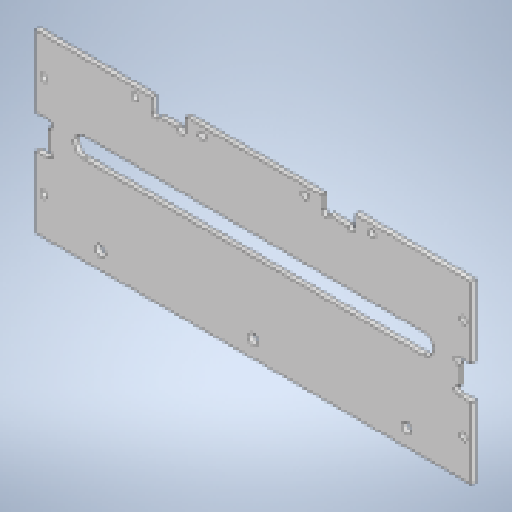
# Autodesk Inventor part: side_ita
Saved by Autodesk Inventor 2024 (Build 280153000, 153)
## iProperties
Created: 2024-06-05
Part Number: side_ita
Material: アルミニウム 2014-T4
Document SubType Name: Modeling
Designer: right
Density: 2.8 g/cm^3
Appearance: サテン
Author: right
Autodesk Inventor part; units mm, degrees
ref_plane "YZ Plane" through (0, 0, 0) normal (1, 0, 0) x (0, 1, 0)
ref_plane "XZ Plane" through (0, 0, 0) normal (0, 1, 0) x (-1, 0, 0)
ref_plane "XY Plane" through (0, 0, 0) normal (0, 0, 1) x (1, 0, 0)
sketch "スケッチ1" plane through (0, 0, 0) normal (0, 0, 1) x (1, 0, 0)
  line L0 (-50.5, 0.75) -> (50.5, 0.75) projected
  line L1 (50.5, 0.75) -> (50.5, 15.0295) projected
  line L2 (50.5, 15.0295) -> (49.637, 17.5) projected
  line L3 (49.637, 17.5) -> (47.2832, 17.5) projected
  line L4 (47.2832, 17.5) -> (44.9252, 10.75) projected
  line L5 (44.9252, 10.75) -> (42.5702, 10.75) projected
  line L6 (42.5702, 10.75) -> (40.2122, 17.5) projected
  line L7 (40.2122, 17.5) -> (37.8584, 17.5) projected
  line L8 (37.8584, 17.5) -> (35.5004, 10.75) projected
  line L9 (35.5004, 10.75) -> (33.1454, 10.75) projected
  line L10 (33.1454, 10.75) -> (30.7874, 17.5) projected
  line L11 (30.7874, 17.5) -> (28.4337, 17.5) projected
  line L12 (28.4337, 17.5) -> (26.0757, 10.75) projected
  line L13 (26.0757, 10.75) -> (23.7207, 10.75) projected
  line L14 (23.7207, 10.75) -> (21.3627, 17.5) projected
  line L15 (21.3627, 17.5) -> (19.0089, 17.5) projected
  line L16 (19.0089, 17.5) -> (16.6509, 10.75) projected
  line L17 (16.6509, 10.75) -> (14.2959, 10.75) projected
  line L18 (14.2959, 10.75) -> (11.9379, 17.5) projected
  line L19 (11.9379, 17.5) -> (9.5841, 17.5) projected
  line L20 (9.5841, 17.5) -> (7.2261, 10.75) projected
  line L21 (7.2261, 10.75) -> (4.8711, 10.75) projected
  line L22 (4.8711, 10.75) -> (2.5131, 17.5) projected
  line L23 (2.5131, 17.5) -> (0.1594, 17.5) projected
  line L24 (0.1594, 17.5) -> (-2.1986, 10.75) projected
  line L25 (-2.1986, 10.75) -> (-4.5536, 10.75) projected
  line L26 (-4.5536, 10.75) -> (-6.9116, 17.5) projected
  line L27 (-6.9116, 17.5) -> (-9.2654, 17.5) projected
  line L28 (-9.2654, 17.5) -> (-11.6234, 10.75) projected
  line L29 (-11.6234, 10.75) -> (-13.9784, 10.75) projected
  line L30 (-13.9784, 10.75) -> (-16.3364, 17.5) projected
  line L31 (-16.3364, 17.5) -> (-18.6902, 17.5) projected
  line L32 (-18.6902, 17.5) -> (-21.0482, 10.75) projected
  line L33 (-21.0482, 10.75) -> (-23.4032, 10.75) projected
  line L34 (-23.4032, 10.75) -> (-25.7612, 17.5) projected
  line L35 (-25.7612, 17.5) -> (-28.115, 17.5) projected
  line L36 (-28.115, 17.5) -> (-30.473, 10.75) projected
  line L37 (-30.473, 10.75) -> (-32.828, 10.75) projected
  line L38 (-32.828, 10.75) -> (-35.186, 17.5) projected
  line L39 (-35.186, 17.5) -> (-37.5397, 17.5) projected
  line L40 (-37.5397, 17.5) -> (-39.8977, 10.75) projected
  line L41 (-39.8977, 10.75) -> (-42.2527, 10.75) projected
  line L42 (-42.2527, 10.75) -> (-44.6107, 17.5) projected
  line L43 (-44.6107, 17.5) -> (-46.9645, 17.5) projected
  line L44 (-46.9645, 17.5) -> (-49.3225, 10.75) projected
  line L45 (-49.3225, 10.75) -> (-50.5, 10.75) projected
  line L46 (-50.5, 10.75) -> (-50.5, 0.75) projected
  circle A0 centre (45.5, 5.75) radius 1.3 projected
  circle A1 centre (0, 5.75) radius 1.1 projected
  circle A2 centre (-45.5, 5.75) radius 1.3 projected
  circle A3 centre (16.0601, 29.9604) radius 1.55 projected
  line L47 (-50.5, 32.9604) -> (50.5, 32.9604)
  line L48 (50.5, 32.9604) -> (50.5, 26.9604)
  line L49 (50.5, 26.9604) -> (-50.5, 26.9604)
  line L50 (-50.5, 26.9604) -> (-50.5, 32.9604)
  circle A4 centre (-50.5, 29.9604) radius 3
  circle A5 centre (50.5, 29.9604) radius 3
  line L51 (-55.5, 52.9604) -> (55.5, 52.9604)
  line L52 (55.5, 52.9604) -> (55.5, 0.75)
  line L53 (55.5, 0.75) -> (-55.5, 0.75)
  line L54 (-55.5, 0.75) -> (-55.5, 52.9604)
  circle A6 centre (-50.5, 29.9604) radius 5 construction
  circle A7 centre (50.5, 29.9604) radius 5 construction
  circle A8 centre (45.5, 5.75) radius 1.6
  circle A9 centre (0, 5.75) radius 1.6
  circle A10 centre (-45.5, 5.75) radius 1.6
  point P0 (0, 0)
  point P1 (0, 52.9604)
  dimension "d0" = 6
  dimension "d1" = 20
  dimension "d2" = 10
  dimension "d3" = 10
  dimension "d6" = 3.2
  dimension "d7" = 3.2
  dimension "d8" = 3.2
  constraints: 16 end point, 6 coincident, 5 centre point, 4 parallel, 3 midpoint, 2 horizontal, 2 perpendicular, 2 tangent, 2 vertical alignment, 1 horizontal alignment, 1 point on line, 6 other
  measures "d0" distance of L49.end L47.start
  measures "d1" distance from line of point (0, 52.96) L47
  measures "d2" diameter of A6
  measures "d3" diameter of A7
  measures "d6" diameter of A8
  measures "d7" diameter of A9
  measures "d8" diameter of A10
extrude "押し出し1" add sketch "スケッチ1" along normal blind 1.5 contours L46 L45 L44 L43 L42 L41 L40 L39 L38 L37 L36 L35 L34 L33 L32 L31 L30 L29 L28 L27 L26 L25 L24 L23 L22 L21 L20 L19 L18 L17 L16 L15 L14 L13 L12 L11 L10 L9 L8 L7 L6 L5 L4 L3 L2 L1 L0 | L53 L54 L51 L52 L1 L2 L3 L4 L5 L6 L7 L8 L9 L10 L11 L12 L13 L14 L15 L16 L17 L18 L19 L20 L21 L22 L23 L24 L25 L26 L27 L28 L29 L30 L31 L32 L33 L34 L35 L36 L37 L38 L39 L40 L41 L42 L43 L44 L45 L46
sketch "スケッチ2" plane through (0, 0, 0) normal (0, 0, -1) x (-1, 0, 0)
  line L0 (-55.5, 0.75) -> (-55.5, 52.9604) projected
  line L1 (55.5, 0.75) -> (-55.5, 0.75) projected
  line L2 (55.5, 52.9604) -> (55.5, 0.75) projected
  line L3 (-55.5, 52.9604) -> (55.5, 52.9604) projected
  circle A0 centre (-45.5, 5.75) radius 1.6 projected
  circle A1 centre (0, 5.75) radius 1.6 projected
  circle A2 centre (45.5, 5.75) radius 1.6 projected
  arc A3 (-50.5, 32.9604) -> (-50.5, 26.9604) centre (-50.5, 29.9604) ccw projected
  line L4 (50.5, 32.9604) -> (-50.5, 32.9604) projected
  arc A4 (50.5, 26.9604) -> (50.5, 32.9604) centre (50.5, 29.9604) ccw projected
  line L5 (-50.5, 26.9604) -> (50.5, 26.9604) projected
  line L6 (-50.5, 48.9435) -> (50.5, 48.9435) construction
  line L7 (50.5, 48.9435) -> (50.5, 51.9435) construction
  line L8 (50.5, 51.9435) -> (-50.5, 51.9435) construction
  line L9 (-50.5, 51.9435) -> (-50.5, 48.9435) construction
  line L10 (0, 50.4435) -> (0, 51.9435) construction
  line L11 (0, 50.4435) -> (-50.5, 50.4435) construction
  line L12 (-30.25, 51.9435) -> (-20.25, 51.9435)
  line L13 (-20.25, 51.9435) -> (-20.25, 48.9435)
  line L14 (-20.25, 48.9435) -> (-30.25, 48.9435)
  line L15 (-30.25, 48.9435) -> (-30.25, 51.9435)
  circle A5 centre (-29.15, 51.9435) radius 1.1
  line L16 (-25.25, 51.9435) -> (-25.25, 50.4435) construction
  circle A6 centre (-21.35, 51.9435) radius 1.1
  circle A7 centre (-29.15, 48.9435) radius 1.1
  circle A8 centre (-21.35, 48.9435) radius 1.1
  circle A9 centre (-35.25, 50.4435) radius 1.1
  line L17 (-101, 51.9435) -> (0, 51.9435) construction
  circle A10 centre (-15.25, 50.4435) radius 1.1
  line L18 (30.25, 51.9435) -> (20.25, 51.9435)
  line L19 (20.25, 51.9435) -> (20.25, 48.9435)
  line L20 (20.25, 48.9435) -> (30.25, 48.9435)
  line L21 (30.25, 48.9435) -> (30.25, 51.9435)
  circle A11 centre (29.15, 51.9435) radius 1.1
  line L22 (25.25, 51.9435) -> (25.25, 50.4435) construction
  circle A12 centre (21.35, 51.9435) radius 1.1
  circle A13 centre (29.15, 48.9435) radius 1.1
  circle A14 centre (21.35, 48.9435) radius 1.1
  circle A15 centre (35.25, 50.4435) radius 1.1
  circle A16 centre (15.25, 50.4435) radius 1.1
  line L23 (-30.25, 51.9435) -> (-30.25, 52.9604)
  line L24 (-20.25, 51.9435) -> (-20.25, 52.9604)
  line L25 (20.25, 51.9435) -> (20.25, 52.9604)
  line L26 (30.25, 51.9435) -> (30.25, 52.9604)
  point P0 (0, 0)
  point P1 (0, 48.9435)
  point P2 (0, 51.1935)
  point P3 (0, 52.9604)
  point P4 (22.45, 48.9435)
  point P5 (28.05, 48.9435)
  point P6 (28.05, 51.9435)
  point P7 (22.45, 51.9435)
  point P8 (20.25, 51.9435)
  point P9 (20.25, 48.9435)
  point P10 (-20.25, 48.9435)
  point P11 (-20.25, 51.9435)
  point P12 (-22.45, 51.9435)
  point P13 (-28.05, 51.9435)
  point P14 (-28.05, 48.9435)
  point P15 (-22.45, 48.9435)
  point P16 (-39.8303, 48.9435)
  point P17 (21.7694, 52.9604)
  point P18 (28.7306, 52.9604)
  point P19 (29.5694, 52.9604)
  point P20 (20.9306, 52.9604)
  point P21 (-20.9306, 52.9604)
  point P22 (-29.5694, 52.9604)
  point P23 (-21.7694, 52.9604)
  point P24 (-28.7306, 52.9604)
  dimension "d13" = 2.2
  dimension "d9" = 3
  dimension "d10" = 5
  dimension "d12" = 10
  dimension "d14" = 2.2
  dimension "d15" = 5
  constraints: 42 end point, 17 symmetric about line, 10 centre point, 10 point on line, 7 midpoint, 7 perpendicular, 4 parallel, 3 horizontal, 3 vertical alignment, 2 vertical, 1 tangent, 16 other
  measures "d9" distance of L8.end L6.start
  measures "d10" distance between parallel lines of L0 L9
  measures "d12" distance between parallel lines of L13 L15
  measures "d14" diameter of A9
  measures "d15" distance from line of L15 A9.centre
extrude "押し出し2" cut sketch "スケッチ2" against normal through all contours L3 A5 L23 | A5 L3 | L3 A5 L12 | A5 L12 A6 L13 A8 L14 A7 L15 | L12 A5 | L26 A11 L3 | L3 A6 L12 A5 | A7 L14 | L14 A7 | A11 L18 L3 | L3 A11 | A11 L18 | L21 A13 L20 A14 L19 A12 L18 A11 | A6 L3 | L3 A6 L12 | L12 A6 | A11 L18 A12 L3 | A13 L20 | L20 A13 | L3 L24 A6 | A8 L14 | L14 A8 | A12 L18 L3 | L3 A12 | A12 L18 | A12 L25 L3 | A14 L20 | L20 A14 | A9 | A10 | A15 | A16
sketch "スケッチ3" plane through (0, 0, 1.5) normal (0, 0, 1) x (1, 0, 0)
  line L0 (60.854, 29.9604) -> (60.854, 48.9604) projected
  line L1 (55.5, 0.75) -> (55.5, 52.9604) projected
  line L2 (55.5, 52.9604) -> (64.854, 52.9604)
  line L3 (64.854, 52.9604) -> (64.854, 0.75)
  line L4 (64.854, 0.75) -> (55.5, 0.75)
  line L5 (55.5, 0.75) -> (55.5, 52.9604)
  line L6 (20.25, 52.9604) -> (-20.25, 52.9604) construction
  line L7 (0, 52.9604) -> (0, 0) construction
  line L8 (-60.854, 29.9604) -> (-60.854, 48.9604)
  line L9 (-55.5, 0.75) -> (-55.5, 52.9604)
  line L10 (-55.5, 52.9604) -> (-64.854, 52.9604)
  line L11 (-64.854, 52.9604) -> (-64.854, 0.75)
  line L12 (-64.854, 0.75) -> (-55.5, 0.75)
  line L13 (-55.5, 0.75) -> (-55.5, 52.9604)
  dimension "d18" = 4
  constraints: 22 end point, 7 symmetric about line, 2 parallel, 2 point on line, 1 horizontal, 1 midpoint, 1 perpendicular, 1 vertical
  measures "d18" distance from line of L0.end L3
extrude "押し出し3" add sketch "スケッチ3" against normal up to surface (1.5 mm away)
sketch "スケッチ4" plane through (0, 0, 0) normal (0, 0, -1) x (-1, 0, 0)
  line L0 (-63.854, 21.8552) -> (-60.854, 21.8552)
  line L1 (-60.854, 21.8552) -> (-60.854, 31.8552)
  line L2 (-60.854, 31.8552) -> (-63.854, 31.8552)
  line L3 (-63.854, 31.8552) -> (-63.854, 21.8552)
  line L4 (-64.854, 52.9604) -> (-64.854, 0.75) projected
  circle A0 centre (-63.854, 22.9552) radius 1.1
  line L5 (-63.854, 21.8552) -> (-64.854, 21.8552)
  circle A1 centre (-63.854, 30.7552) radius 1.1
  line L6 (-63.854, 31.8552) -> (-64.854, 31.8552)
  line L7 (-62.354, 31.8552) -> (-62.354, 21.8552) construction
  circle A2 centre (-60.854, 22.9552) radius 1.1
  circle A3 centre (-60.854, 30.7552) radius 1.1
  line L8 (-63.854, 26.8552) -> (-60.854, 26.8552) construction
  circle A4 centre (-62.354, 41.8552) radius 1.1
  circle A5 centre (-62.354, 41.8552) radius 1.1
  circle A6 centre (-62.354, 11.8552) radius 1.1
  line L9 (-20.25, 52.9604) -> (20.25, 52.9604) construction
  line L10 (0, 52.9604) -> (0, 0) construction
  line L11 (63.854, 21.8552) -> (60.854, 21.8552)
  line L12 (60.854, 21.8552) -> (60.854, 31.8552)
  line L13 (60.854, 31.8552) -> (63.854, 31.8552)
  line L14 (63.854, 31.8552) -> (63.854, 21.8552)
  line L15 (64.854, 52.9604) -> (64.854, 0.75)
  circle A7 centre (63.854, 22.9552) radius 1.1
  line L16 (63.854, 21.8552) -> (64.854, 21.8552)
  circle A8 centre (63.854, 30.7552) radius 1.1
  line L17 (63.854, 31.8552) -> (64.854, 31.8552)
  line L18 (62.354, 31.8552) -> (62.354, 21.8552) construction
  circle A9 centre (60.854, 22.9552) radius 1.1
  circle A10 centre (60.854, 30.7552) radius 1.1
  line L19 (63.854, 26.8552) -> (60.854, 26.8552) construction
  circle A11 centre (62.354, 41.8552) radius 1.1
  circle A12 centre (62.354, 41.8552) radius 1.1
  circle A13 centre (62.354, 11.8552) radius 1.1
  point P0 (-64.854, 26.8552)
  point P1 (-64.854, 31.2135)
  point P2 (-64.854, 30.2969)
  point P3 (-64.854, 23.4135)
  point P4 (-64.854, 22.4969)
  point P5 (-60.854, 24.0552)
  point P6 (-60.854, 29.6552)
  point P7 (64.854, 26.8552)
  point P8 (64.854, 30.2969)
  point P9 (64.854, 31.2135)
  point P10 (60.854, 29.6552)
  point P11 (60.854, 24.0552)
  point P12 (64.854, 22.4969)
  point P13 (64.854, 23.4135)
  dimension "d24" = 2.2
  dimension "d21" = 3
  dimension "d22" = 10
  dimension "d23" = 4
  dimension "d25" = 2.2
  dimension "d26" = 10
  constraints: 36 end point, 22 symmetric about line, 10 centre point, 8 point on line, 6 midpoint, 3 perpendicular, 3 vertical, 2 horizontal, 2 parallel, 1 horizontal alignment, 1 vertical alignment, 21 other
  measures "d21" distance of L2.end L1.end
  measures "d22" distance of L1.end L0.end
  measures "d23" distance between parallel lines of L4 L1
  measures "d25" diameter of A4
  measures "d26" distance from line of L2 A4.centre
extrude "押し出し4" cut sketch "スケッチ4" against normal through all
